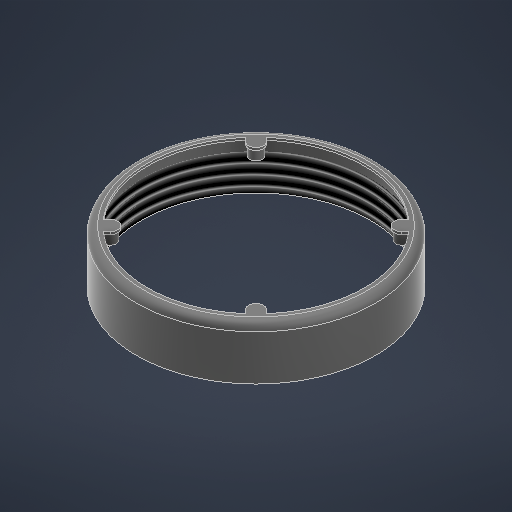
# Autodesk Inventor part: DisplayCover
Saved by Autodesk Inventor 2026.2 (Build 302298000, 298)
## iProperties
Created: 2026-06-05
Part Number: DisplayCover
Material: Generic
Document SubType Name: Modeling
Designer: User
Density: 1 g/cm^3
Appearance: Default
Author: User
Autodesk Inventor part; units mm, degrees
ref_plane "YZ Plane" through (0, 0, 0) normal (1, 0, 0) x (0, 1, 0)
ref_plane "XZ Plane" through (0, 0, 0) normal (0, 1, 0) x (-1, 0, 0)
ref_plane "XY Plane" through (0, 0, 0) normal (0, 0, 1) x (1, 0, 0)
sketch "Sketch1" plane through (0, 0, 0) normal (0, 1, 0) x (-1, 0, 0)
  circle A0 centre (0, 0) radius 45 construction
  circle A1 centre (0, 0) radius 47.5
  circle A2 centre (29, 29) radius 1.5 construction
  circle A3 centre (29, 29) radius 3 construction
  arc A4 (26.8787, 31.1213) -> (31.1213, 26.8787) centre (29, 29) ccw
  line L0 (26.8787, 31.1213) -> (28.2102, 32.4528)
  line L1 (31.1213, 26.8787) -> (32.4528, 28.2102)
  circle A5 centre (-29, 29) radius 1.5 construction
  circle A6 centre (-29, 29) radius 3 construction
  line L2 (-31.1213, 26.8787) -> (-32.4528, 28.2102)
  line L3 (-26.8787, 31.1213) -> (-28.2102, 32.4528)
  arc A7 (-31.1213, 26.8787) -> (-26.8787, 31.1213) centre (-29, 29) ccw
  circle A8 centre (-29, -29) radius 1.5 construction
  circle A9 centre (-29, -29) radius 3 construction
  line L4 (-26.8787, -31.1213) -> (-28.2102, -32.4528)
  line L5 (-31.1213, -26.8787) -> (-32.4528, -28.2102)
  arc A10 (-26.8787, -31.1213) -> (-31.1213, -26.8787) centre (-29, -29) ccw
  circle A11 centre (29, -29) radius 1.5 construction
  circle A12 centre (29, -29) radius 3 construction
  line L6 (31.1213, -26.8787) -> (32.4528, -28.2102)
  line L7 (26.8787, -31.1213) -> (28.2102, -32.4528)
  arc A13 (31.1213, -26.8787) -> (26.8787, -31.1213) centre (29, -29) ccw
  arc A14 (32.4528, -28.2102) -> (32.4528, 28.2102) centre (0, 0) ccw
  arc A15 (-28.2102, -32.4528) -> (28.2102, -32.4528) centre (0, 0) ccw
  arc A16 (28.2102, 32.4528) -> (-28.2102, 32.4528) centre (0, 0) ccw
  arc A17 (-32.4528, 28.2102) -> (-32.4528, -28.2102) centre (0, 0) ccw
  dimension "d0" = 90
  dimension "d3" = 2.5
  dimension "d6" = 3
  dimension "d7" = 29
  dimension "d8" = 29
  dimension "d9" = 1.5
  dimension "d16" = 360
  dimension "d18" = 2
  constraints: 18 centre point, 16 end point, 16 point on circle, 5 coincident, 4 tangent, 2 parallel, 1 concentric, 45 other
  measures "d0" diameter of A0
  measures "d3" radial gap between concentric circles of A0 A1
  measures "d6" diameter of A2
  measures "d7" horizontal distance of point (0, 0) A2.centre
  measures "d8" horizontal distance of point (0, 0) A2.centre
  measures "d9" radial gap between concentric circles of A3 A2
  measures "d18" radial gap between concentric circles of A0 A17
extrude "Ring" add sketch "Sketch1" against normal blind 1
sketch "Sketch2" plane through (0, -1, 0) normal (0, -1, 0) x (-1, 0, 0)
  circle A0 centre (-29, -29) radius 1.5 construction
  circle A1 centre (-29, -29) radius 2.5
  circle A2 centre (29, -29) radius 2.5
  circle A3 centre (29, 29) radius 2.5
  circle A4 centre (-29, 29) radius 2.5
  circle A5 centre (29, 29) radius 1.5 construction
  circle A6 centre (-29, 29) radius 1.5 construction
  circle A7 centre (29, -29) radius 1.5 construction
  circle A8 centre (-29, -29) radius 1.5
  circle A9 centre (29, -29) radius 1.5
  circle A10 centre (29, 29) radius 1.5
  circle A11 centre (-29, 29) radius 1.5
  point P0 (0, 0)
  dimension "d19" = 1
  dimension "d22" = 360
  constraints: 8 centre point, 4 coincident, 4 concentric, 9 other
  measures "d19" radial gap between concentric circles of A1 A0
extrude "BoardHolder" add sketch "Sketch2" along normal blind 4
sketch "Sketch3" plane through (0, -1, 0) normal (0, -1, 0) x (1, 0, 0)
  circle A0 centre (0, 0) radius 45.5
  circle A1 centre (0, 0) radius 47.5
  circle A2 centre (0, 0) radius 47.5 projected
  dimension "d26" = 91
  constraints: 2 centre point, 2 coincident, 1 concentric
  measures "d26" diameter of A0
extrude "Extrusion3" add sketch "Sketch3" along normal blind 20
fillet "Fillet1" radius 3 1 edges at (47.5, 0, 0)
thread "Thread1" size "M95x4" class "6H" standard "ISO Metric profile" length 14.4 offset 5.6
body "Solid1"
